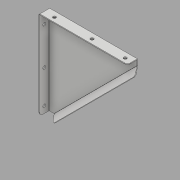
# Autodesk Inventor part: 2-4-1
Saved by Autodesk Inventor 2019 (Build 230136000, 136)
## iProperties
Part Number: 2-4-1
Material: 一般
Document SubType Name: Modeling
Designer: d8910
Density: 1 g/cm^3
Appearance: 預設
Author: d8910
Autodesk Inventor part; units mm, degrees
ref_plane "YZ Plane" through (0, 0, 0) normal (1, 0, 0) x (0, 1, 0)
ref_plane "XZ Plane" through (0, 0, 0) normal (0, 1, 0) x (-1, 0, 0)
ref_plane "XY Plane" through (0, 0, 0) normal (0, 0, 1) x (1, 0, 0)
sketch "草圖1" plane through (0, 0, 0) normal (0, 1, 0) x (-1, 0, 0)
  line L0 (0, 0) -> (0, -200)
  line L1 (0, -200) -> (200, 0) construction
  line L2 (200, 0) -> (0, 0)
  line L3 (13.5, -200) -> (13.5, -13.5) construction
  line L4 (13.5, -13.5) -> (200, -13.5) construction
  line L5 (200, 0) -> (200, -13.5)
  line L6 (0, -200) -> (13.5, -200)
  line L7 (200, -13.5) -> (13.5, -200)
  dimension "d0" = 200
  dimension "d1" = 13.5
  dimension "d2" = 13.5
  constraints: 16 end point, 4 perpendicular, 2 vertical
  measures "d0" distance of L1.end L0.start
  measures "d1" distance between parallel lines of L2 L4
  measures "d2" distance between parallel lines of L0 L3
extrude "擠出1" add sketch "草圖1" along normal blind 2
sketch "草圖2" plane through (0, 2, 0) normal (0, 1, 0) x (1, 0, 0)
  line L0 (-200, 13.5) -> (-200, 0) construction
  line L1 (0, 0) -> (0, 200) projected
  line L2 (-200, 0) -> (0, 0)
  line L3 (0, 0) -> (0, 4.6333)
  line L4 (-2, 2) -> (-200, 2)
  line L5 (-200, 2) -> (-200, 0)
  line L6 (-200, 0) -> (0, 0) projected
  line L7 (0, 200) -> (-2, 200)
  line L8 (-2, 200) -> (-2, 2)
  line L9 (-4.9528, 0) -> (0, 0)
  line L10 (0, 0) -> (0, 200)
  line L11 (-2, 0) -> (-2, 2)
  line L12 (-2, 2) -> (0, 2)
  dimension "d5" = 2
  dimension "d6" = 2
  constraints: 20 end point, 4 parallel, 4 point on line, 3 perpendicular, 2 horizontal, 1 vertical
  measures "d5" distance of L1.end L7.end
  measures "d6" distance from line of L2 L4.end
extrude "擠出2" add sketch "草圖2" along normal blind 21
sketch "草圖3" plane through (0, 23, 0) normal (0, 1, 0) x (1, 0, 0)
  line L0 (-2, 200) -> (-2, 2) projected
  line L1 (-2, 2) -> (0, 2)
  line L2 (0, 2) -> (0, 0)
  line L3 (0, 0) -> (-2, 0)
  line L4 (-2, 0) -> (-2, 2)
  constraints: 8 end point, 2 parallel, 1 horizontal, 1 perpendicular
extrude "擠出3" cut sketch "草圖3" against normal through all
fillet "圓角1" radius 0.74 2 edges at (-101, 0, 0) (0, 0, -101)
sketch "草圖4" plane through (0, 2, 0) normal (0, 1, 0) x (1, 0, 0)
  line L0 (-123.1874, -123.1874) -> (134.1745, 134.1745)
  line L1 (-200, 0) -> (-2, 0) projected
  point P0 (0, 0)
  dimension "d12" = 45
  constraints: 2 end point, 1 point on line
  measures "d12" angle of L0 L1
surface extrude "擠出表面1" sketch "草圖4" along normal blind 254.25 shown no curves L0
sketch "草圖9" plane through (-2, 23, 0) normal (1, 0, 0) x (0, 0, -1)
  arc A0 (0, -22.26) -> (0.74, -23) centre (0.74, -22.26) ccw construction
  line L0 (2, -23) -> (0.74, -23) construction
  line L1 (2, -21) -> (2, -23) construction
  line L2 (2, 0) -> (2, -21) construction
  line L3 (0, 0) -> (2, 0) construction
  line L4 (0, -22.26) -> (0, 0) construction
  line L5 (2, 0) -> (2, -21) projected
  point P0 (0, -23)
  point P1 (2, -18.4491)
  constraints: 1 point on line
sketch "草圖8" plane through (0, 0, 0) normal (0, -1, 0) x (1, 0, 0)
  line L0 (0, 0) -> (-2.1509, -2.1509) construction
  arc A0 (-1.2239, -2) -> (-2.1509, -2.1509) centre (-1.2239, -4.923) ccw
  arc A1 (-2.1509, -2.1509) -> (-2, -1.2239) centre (-4.923, -1.2239) ccw
  line L1 (-0.74, -2) -> (-2, -2) construction
  arc A2 (-2, -1.2239) -> (-1.2239, -2) centre (-1.2239, -1.2239) ccw
  line L2 (-2, -2) -> (-2, -0.74) construction
  constraints: 6 point on circle, 3 centre point, 2 end point, 2 point on line, 2 symmetric about line, 2 tangent, 1 other
loft "斷面混成1" cut profiles "草圖8" section 2 point at (-2, 4.5509, -2)
sketch "草圖10" plane through (-200, 0, -13.5) normal (-1, 0, 0) x (0, 0, 1)
  arc A0 (12.76, 0) -> (13.5, 0.74) centre (12.76, 0.74) ccw construction
  line L0 (13.5, 0.74) -> (13.5, 23) construction
  line L1 (11.5, 23) -> (13.5, 23) construction
  line L2 (11.5, 2) -> (11.5, 23) construction
  line L3 (0, 2) -> (11.5, 2) construction
  line L4 (0, 0) -> (0, 2) construction
  line L5 (0, 0) -> (12.76, 0) construction
  line L6 (11.4412, 2) -> (-186.5, 2) construction
  arc A1 (10.76, 2) -> (11.5, 2.74) centre (10.76, 2.74) ccw
  line L7 (0, 2) -> (11.5, 2) construction
  line L8 (11.5, 2) -> (11.5, 23) construction
  line L9 (11.5, 2) -> (11.4154, 2) projected
  line L10 (10.76, 2) -> (11.5, 2)
  line L11 (11.5, 2) -> (11.5, 2.74)
  point P0 (13.5, 0)
  dimension "d23" = 0.74
  constraints: 4 end point, 3 tangent, 2 point on circle, 2 point on line, 1 centre point, 1 horizontal, 1 perpendicular
  measures "d23" radius of A1
sketch "草圖11" plane through (0, 2, 0) normal (0, 1, 0) x (1, 0, 0)
  line L0 (-200, 2) -> (-2.0588, 2) projected
  line L1 (-200, 2) -> (-2.0588, 2)
  point P0 (0, 0)
  constraints: 2 end point, 1 horizontal
sketch3d "3D 草圖1"
  line L0 (-200, 2, -2) -> (-2.0588, 2, -2)
sweep "掃掠1" add profiles "草圖10" path "3D 草圖1"
sketch "草圖12" plane through (-13.5, 0, -200) normal (0, 0, -1) x (-1, 0, 0)
  arc A0 (-13.5, 0.74) -> (-12.76, 0) centre (-12.76, 0.74) ccw construction
  line L0 (-12.76, 0) -> (0, 0) construction
  line L1 (0, 0) -> (0, 2) construction
  line L2 (-11.5, 2) -> (0, 2) construction
  line L3 (-11.5, 2) -> (-11.5, 23) construction
  line L4 (-13.5, 23) -> (-11.5, 23) construction
  line L5 (-13.5, 0.74) -> (-13.5, 23) construction
  arc A1 (-11.5, 2.74) -> (-10.76, 2) centre (-10.76, 2.74) ccw
  line L6 (-11.5, 2.74) -> (-11.5, 2)
  line L7 (-11.5, 4.5509) -> (-11.5, 0) projected
  line L8 (-11.5, 2) -> (0, 2) projected
  line L9 (-10.76, 2) -> (-11.5, 2)
  point P0 (-13.5, 0)
  dimension "d26" = 0.74
  constraints: 4 end point, 3 tangent, 2 collinear, 2 point on circle, 2 point on line, 1 centre point
  measures "d26" radius of A1
sketch "草圖13" plane through (0, 2, 0) normal (0, 1, 0) x (1, 0, 0)
  line L0 (-2, 2.0588) -> (-2, 2) projected
  line L1 (-2, 2.0588) -> (-2, 200) projected
  line L2 (-2, 2.0588) -> (-2, 200)
  point P0 (0, 0)
  constraints: 2 end point, 1 vertical
sketch3d "3D 草圖2"
  line L0 (-2, 2, -200) -> (-2, 2, -2.0588)
sweep "掃掠2" add profiles "草圖12" path "3D 草圖2"
loft "斷面混成2" cut profiles "草圖8" section 1 point at (-2, 4.5509, -2)
delete faces "刪除面1" heal yes whole lump no faces at (-2.0588, 2.3602, -2.0191)
delete faces "刪除面2" heal yes whole lump no faces at (-2.0191, 2.3602, -2.0588)
sketch "草圖14" plane through (-2.0417, 2.74, -2) normal (0, 0, -1) x (-1, 0, 0)
  line L0 (0, 0) -> (197.9583, 0) construction
  line L1 (197.9583, 0) -> (197.9583, 20.26) construction
  line L2 (-0.0417, 20.26) -> (197.9583, 20.26) construction
  line L3 (-0.0417, 20.26) -> (-0.0417, 1.8109) construction
  line L4 (-0.0417, 1.8109) -> (0, 0) construction
  circle A0 centre (22.9583, 10.26) radius 3.5
  circle A1 centre (107.9583, 10.26) radius 3.5
  circle A2 centre (182.9583, 10.26) radius 3.5
  point P0 (-2.0417, -2.74)
  dimension "d33" = 10
  dimension "d34" = 7
  dimension "d35" = 15
  dimension "d36" = 75
  dimension "d37" = 85
  constraints: 3 centre point, 2 equal radius, 2 horizontal alignment
  measures "d33" distance from line of L2 A2.centre
  measures "d34" diameter of A2
  measures "d35" distance from line of L1 A2.centre
  measures "d36" distance of A1.centre A2.centre
  measures "d37" distance of A1.centre A0.centre
extrude "擠出4" cut sketch "草圖14" against normal blind 10
fillet "圓角2" radius 6 1 edges at (-200, 23, -1)
fillet "圓角3" radius 6 1 edges at (-1, 23, -200)
sketch "草圖15" plane through (-2, 4.5509, -2) normal (-1, 0, 0) x (0, 0, 1)
  circle A0 centre (-183, 8.4491) radius 3.5
  circle A1 centre (-108, 8.4491) radius 3.5
  circle A2 centre (-23, 8.4491) radius 3.5
  line L0 (-198, -1.8109) -> (-198, 12.4491) projected
  line L1 (-192, 18.4491) -> (0, 18.4491) projected
  point P0 (2, -4.5509)
  dimension "d42" = 7
  dimension "d43" = 15
  dimension "d44" = 75
  dimension "d45" = 85
  dimension "d46" = 10
  constraints: 3 centre point, 2 equal radius, 2 horizontal alignment
  measures "d42" diameter of A2
  measures "d43" distance from line of L0 A0.centre
  measures "d44" distance of A1.centre A0.centre
  measures "d45" distance of A1.centre A2.centre
  measures "d46" distance from line of L1 A0.centre
extrude "擠出5" cut sketch "草圖15" against normal through all
sketch "草圖16" plane through (0, 2, 0) normal (0, 1, 0) x (1, 0, 0)
  line L0 (-2.74, 200) -> (-13.5, 200) construction
  line L1 (-13.5, 200) -> (-25.4459, 211.9459)
  line L2 (-13.5, 200) -> (-200, 13.5) construction
  point P0 (0, 0)
  constraints: 2 end point, 1 perpendicular
surface extrude "擠出表面4" sketch "草圖16" along normal blind 23.25 shown no curves L1
sketch "草圖17" plane through (-13.5, 2, -200) normal (-0.7071068, 0, 0.7071068) x (0.7071068, 0, 0.7071068)
  line L0 (0, -2) -> (9.0227, -2) projected
  line L1 (0, -2) -> (-13.7279, 11.7279)
  line L2 (0, 0) -> (7.6085, 0) projected
  line L3 (0, 0) -> (-12.7279, 12.7279)
  line L4 (0, -2) -> (0, 0) projected
  line L5 (-12.7279, 12.7279) -> (-13.7279, 11.7279)
  point P0 (150.9673, -2)
  dimension "d51" = 18
  dimension "d52" = 135
  constraints: 6 end point, 1 parallel, 1 perpendicular
  measures "d51" distance of L3.end L2.start
  measures "d52" angle of L2 L3
sketch "草圖18" plane through (0, 2, 0) normal (0, 1, 0) x (1, 0, 0)
  line L0 (-13.5, 200) -> (-200, 13.5) projected
  point P0 (0, 0)
sweep "掃掠3" add profiles "草圖17" path "草圖18"
fillet "圓角4" radius 0.5 2 edges at (-106.75, 0, -106.75) (-106.75, 2, -106.75)
fillet "圓角5" radius 6 2 edges at (-22.8536, 14.2279, -209.3536) (-209.3536, 14.2279, -22.8536)
